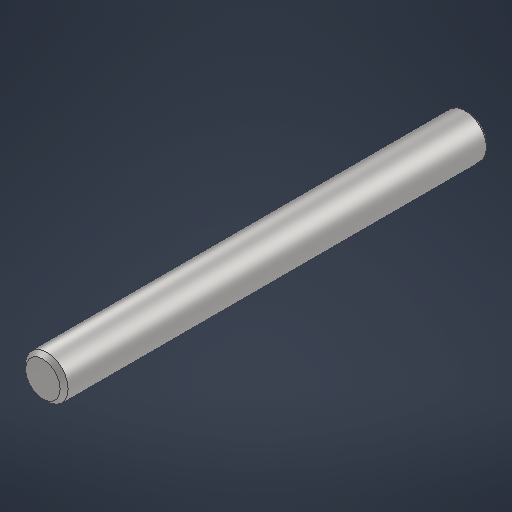
# Autodesk Inventor part: Part10
Saved by Autodesk Inventor 2026 (Build 300175000, 175)
## iProperties
Created: 2026-03-22
Part Number: Part10
Material: Generic
Document SubType Name: Modeling
Designer: Mlinč
Density: 1 g/cm^3
Appearance: Default
Author: Mlinč
Autodesk Inventor part; units mm, degrees
ref_plane "YZ Plane" through (0, 0, 0) normal (1, 0, 0) x (0, 1, 0)
ref_plane "XZ Plane" through (0, 0, 0) normal (0, 1, 0) x (-1, 0, 0)
ref_plane "XY Plane" through (0, 0, 0) normal (0, 0, 1) x (1, 0, 0)
sketch "Sketch1" plane through (0, 0, 0) normal (0, 0, 1) x (1, 0, 0)
  circle A0 centre (0, 0) radius 4
  dimension "d0" = 8
  constraints: 1 centre point, 1 coincident
  measures "d0" diameter of A0
extrude "Extrusion1" add sketch "Sketch1" against normal blind 80
chamfer "Chamfer1" distance 0.75 angle 45 2 edges at (-4, 0, 0) (-4, 0, -80)
body "Solid1"
